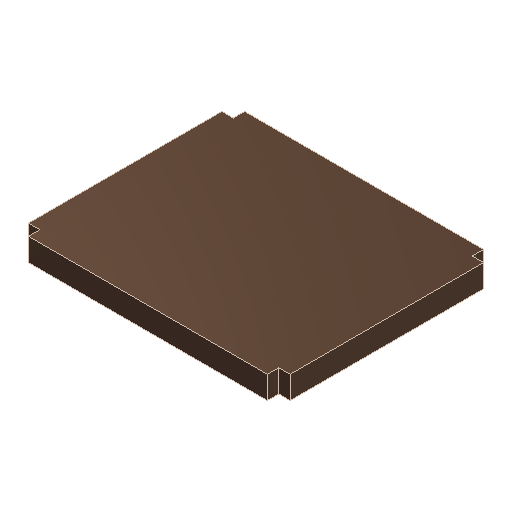
# Autodesk Inventor part: cover__1
Saved by Autodesk Inventor 2025.2 (Build 292293000, 293)
## iProperties
Created: 2025-03-28
Part Number: cover__1
Material: 청동, 주조
Document SubType Name: Modeling
Designer: jbhma
Density: 8.87 g/cm^3
Appearance: 청동 - 새틴
Author: jbhma
Autodesk Inventor part; units mm, degrees
ref_plane "YZ Plane" through (0, 0, 0) normal (1, 0, 0) x (0, 1, 0)
ref_plane "XZ Plane" through (0, 0, 0) normal (0, 1, 0) x (-1, 0, 0)
ref_plane "XY Plane" through (0, 0, 0) normal (0, 0, 1) x (1, 0, 0)
sketch "스케치1" plane through (0, 0, 0) normal (0, 1, 0) x (-1, 0, 0)
  line L0 (0, 0) -> (-420, 0)
  line L1 (-420, 0) -> (-420, -340)
  line L2 (-420, -340) -> (0, -340)
  line L3 (0, -340) -> (0, 0)
  line L4 (0, 0) -> (-420, 0)
  line L5 (0, -340) -> (-420, -340)
  line L6 (-420, -340) -> (-420, -360)
  line L7 (-420, -360) -> (0, -360)
  line L8 (0, -360) -> (0, -340)
  line L9 (0, 0) -> (20, 0)
  line L10 (20, 0) -> (20, -340)
  line L11 (20, -340) -> (0, -340)
  line L12 (0, -340) -> (0, 0)
  line L13 (-420, 0) -> (-440, 0)
  line L14 (-440, 0) -> (-440, -340)
  line L15 (-440, -340) -> (-420, -340)
  line L16 (-420, -340) -> (-420, 0)
  line L17 (0, 0) -> (-420, 0)
  line L18 (-420, 0) -> (-420, 20)
  line L19 (-420, 20) -> (0, 20)
  line L20 (0, 20) -> (0, 0)
  dimension "d0" = 420
  dimension "d1" = 340
  dimension "d2" = 20
  dimension "d3" = 20
  dimension "d4" = 340
  dimension "d5" = 20
  dimension "d6" = 20
  constraints: 42 end point, 10 parallel, 6 horizontal, 5 perpendicular, 1 point on line
  measures "d0" distance of L2.end L1.end
  measures "d1" distance of L1.end L0.end
  measures "d2" distance of L6.end L5.end
  measures "d3" distance of L10.end L11.end
  measures "d4" distance of L9.end L10.end
  measures "d5" distance of L15.end L14.end
  measures "d6" distance of L17.end L18.end
extrude "돌출3" add sketch "스케치1" along normal blind 20
sketch "스케치3" plane through (0, 0, 0) normal (0, -1, 0) x (1, 0, 0)
  line L0 (0, 0) -> (420, 0)
  line L1 (420, 0) -> (420, 20)
  line L2 (420, 20) -> (0, 20)
  line L3 (0, 20) -> (0, 0)
  line L4 (420, 0) -> (440, 0)
  line L5 (440, 0) -> (440, -340)
  line L6 (440, -340) -> (420, -340)
  line L7 (420, -340) -> (420, 0)
  line L8 (420, -340) -> (0, -340)
  line L9 (0, -340) -> (0, -360)
  line L10 (0, -360) -> (420, -360)
  line L11 (420, -360) -> (420, -340)
  line L12 (0, -340) -> (-20, -340)
  line L13 (-20, -340) -> (-20, 0)
  line L14 (-20, 0) -> (0, 0)
  line L15 (0, 0) -> (0, -340)
  constraints: 32 end point, 8 parallel, 4 horizontal, 4 perpendicular, 2 point on line
extrude "돌출4" add sketch "스케치3" along normal blind 20 contours L3 L2 L1 L0 | L15 L12 L13 L14 | L4 L5 L6 L7 | L8 L11 L10 L9
